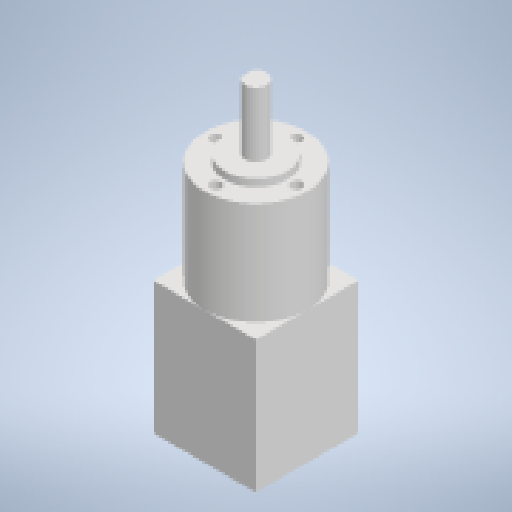
# Autodesk Inventor part: 28stepper27
Saved by Autodesk Inventor 2025 (Build 290162000, 162)
## iProperties
Created: 2025-07-04
Part Number: 28stepper27
Material: 一般
Document SubType Name: Modeling
Designer: gavin
Density: 1 g/cm^3
Appearance: 預設
Author: gavin
Autodesk Inventor part; units mm, degrees
ref_plane "YZ Plane" through (0, 0, 0) normal (1, 0, 0) x (0, 1, 0)
ref_plane "XZ Plane" through (0, 0, 0) normal (0, 1, 0) x (-1, 0, 0)
ref_plane "XY Plane" through (0, 0, 0) normal (0, 0, 1) x (1, 0, 0)
sketch "草圖1" plane through (0, 0, 0) normal (0, 1, 0) x (-1, 0, 0)
  line L0 (14, 14) -> (-14, 14)
  line L1 (-14, 14) -> (-14, -14)
  line L2 (-14, -14) -> (14, -14)
  line L3 (14, -14) -> (14, 14)
  line L4 (14, 14) -> (-14, -14) construction
  line L5 (-14, 14) -> (14, -14) construction
  point P0 (0, 0)
  dimension "d0" = 28
  dimension "d1" = 28
  constraints: 12 end point, 2 midpoint, 2 parallel, 1 horizontal, 1 perpendicular
  measures "d0" distance of L2.end L1.end
  measures "d1" distance of L1.end L0.end
extrude "擠出1" add sketch "草圖1" along normal blind 36
sketch "草圖2" plane through (0, 36, 0) normal (0, 1, 0) x (1, 0, 0)
  circle A0 centre (0, 0) radius 14
  constraints: 1 centre point, 1 coincident
extrude "擠出2" add sketch "草圖2" along normal blind 28
sketch "草圖3" plane through (0, 64, 0) normal (0, 1, 0) x (1, 0, 0)
  circle A0 centre (0, 0) radius 8.5
  dimension "d6" = 17
  constraints: 1 centre point, 1 coincident
  measures "d6" diameter of A0
extrude "擠出3" add sketch "草圖3" along normal blind 2
sketch "草圖4" plane through (0, 66, 0) normal (0, 1, 0) x (1, 0, 0)
  circle A0 centre (0, 0) radius 3
  dimension "d9" = 6
  constraints: 1 centre point, 1 coincident
  measures "d9" diameter of A0
extrude "擠出4" add sketch "草圖4" along normal blind 17.5
sketch "草圖5" plane through (0, 83.5, 0) normal (0, 1, 0) x (1, 0, 0)
  circle A0 centre (0, 0) radius 3 projected
  line L0 (-2.5, -1.6583) -> (-2.5, 1.6583)
  point P0 (3, 0)
  dimension "d13" = 5.5
  constraints: 3 point on circle, 2 end point, 1 vertical
  measures "d13" distance from line of A0.start L0
extrude "擠出5" cut sketch "草圖5" against normal blind 15 contours L0 A0 picked at (-2.6056, 0.3442)
sketch "草圖6" plane through (0, 64, 0) normal (0, 1, 0) x (1, 0, 0)
  circle A0 centre (0, 0) radius 11
  circle A1 centre (0, 11) radius 1.5
  circle A2 centre (-11, 0) radius 1.5
  circle A3 centre (0, -11) radius 1.5
  circle A4 centre (11, 0) radius 1.5
  dimension "d16" = 22
  dimension "d17" = 3
  dimension "d20" = 360
  constraints: 4 centre point, 1 coincident, 1 vertical alignment, 11 other
  measures "d17" diameter of A1
extrude "擠出6" cut sketch "草圖6" against normal blind 10 contours A0 A4 | A0 A4 | A1 A0 | A0 A1 | A3 A0 | A0 A3 | A2 A0 | A0 A2
